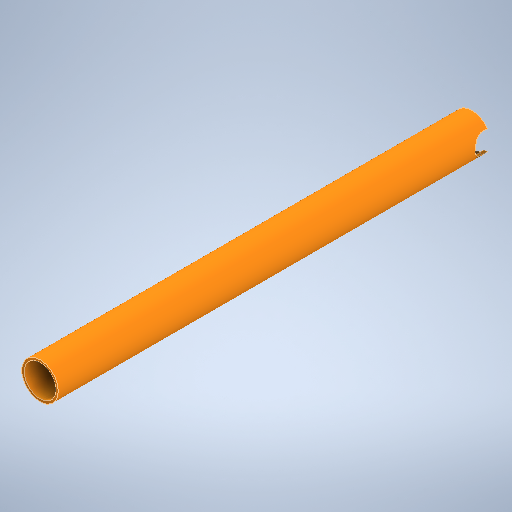
# Autodesk Inventor part: 132 part 1
Saved by Autodesk Inventor 2025.1 (Build 291241000, 241)
## iProperties
Created: 2024-08-01
Part Number: 132 part 1
Material: Aluminum 6061-AHC
Document SubType Name: Modeling
Designer: ffogue
Density: 2.7 g/cm^3
Appearance: Orange
Author: ffogue
Autodesk Inventor part; units mm, degrees
ref_plane "XZ Plane" through (0, 0, 0) normal (0, 1, 0) x (-1, 0, 0)
ref_plane "XY Plane" through (0, 0, 0) normal (0, 0, 1) x (1, 0, 0)
sketch "Sketch1" plane through (0, 0, 0) normal (0, 0, 1) x (1, 0, 0)
  line L0 (0, 0) -> (0, 260)
  line L1 (0, 260) -> (11, 260)
  line L2 (11, 260) -> (11, 0)
  line L3 (11, 0) -> (0, 0)
  dimension "d0" = 22
  dimension "d1" = 260
  constraints: 8 end point, 3 perpendicular, 1 vertical
  measures "d0" diameter of L2 L0
  measures "d1" distance of L0.start L0.end
revolve "Revolution1" add sketch "Sketch1" angle 360 about axis through (0, 0, 0) along (0, 1, 0)
sketch "Sketch2" plane through (0, 0, 0) normal (0, -1, 0) x (1, 0, 0)
  circle A0 centre (0, 0) radius 11 projected
  constraints: 1 coincident
hole "Hole1" at (0, 0, 0) direction (0, 1, 0) diameter 19 depth 260
ref_plane "Work Plane1" through (11, 0, 0) normal (1, 0, 0) x (0, 1, 0)
sketch "Sketch3" plane through (11, 0, 0) normal (1, 0, 0) x (0, 1, 0)
  line L0 (260, -11) -> (260, 11) projected
  line L1 (0, -11) -> (0, 11) projected
  line L2 (0, -11) -> (260, -11) projected
  line L3 (0, 11) -> (260, 11) projected
  line L4 (260, -6) -> (257, -6)
  arc A0 (257, 6) -> (257, -6) centre (257, 0) ccw
  line L5 (257, 6) -> (260, 6)
  point P0 (0, 0)
  point P1 (0, 0)
  dimension "d11" = 3
  dimension "d12" = 6
  constraints: 4 end point, 2 point on circle, 2 point on line, 2 tangent, 1 centre point, 1 horizontal, 1 horizontal alignment, 1 midpoint, 1 perpendicular
  measures "d11" distance from line of L0 A0.centre
  measures "d12" radius of A0
extrude "Extrusion1" cut sketch "Sketch3" against normal up to surface contours L4 A0 L5 L0
body "Solid1"
